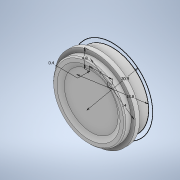
# Autodesk Inventor part: fingerprint sensor
Saved by Autodesk Inventor 2022 (Build 260153000, 153)
## iProperties
Created: 2022-06-08
Part Number: fingerprint sensor
Material: Generic
Document SubType Name: Modeling
Designer: alecw
Density: 1 g/cm^3
Appearance: Default
Author: alecw
Autodesk Inventor part; units mm, degrees
ref_plane "YZ Plane" through (0, 0, 0) normal (1, 0, 0) x (0, 1, 0)
ref_plane "XZ Plane" through (0, 0, 0) normal (0, 1, 0) x (-1, 0, 0)
ref_plane "XY Plane" through (0, 0, 0) normal (0, 0, 1) x (1, 0, 0)
sketch "Sketch1" plane through (0, 0, 0) normal (0, 0, 1) x (1, 0, 0)
  circle A0 centre (0, 0) radius 9.4
  circle A1 centre (0, 0) radius 10.45
  circle A2 centre (0, 0) radius 7
  line L0 (0, 0) -> (0, 1)
  line L1 (0, 1) -> (-5.6, 1)
  line L2 (-6, 1.4) -> (-6, 5.4)
  line L3 (-5.6, 5.8) -> (0, 5.8)
  arc A3 (-6, 1.4) -> (-5.6, 1) centre (-5.6, 1.4) ccw
  arc A4 (-5.6, 5.8) -> (-6, 5.4) centre (-5.6, 5.4) ccw
  line L4 (0, 1) -> (5.6, 1)
  line L5 (6, 1.4) -> (6, 5.4)
  line L6 (5.6, 5.8) -> (0, 5.8)
  arc A5 (5.6, 1) -> (6, 1.4) centre (5.6, 1.4) ccw
  arc A6 (6, 5.4) -> (5.6, 5.8) centre (5.6, 5.4) ccw
  point P0 (-6, 1)
  point P1 (-6, 5.8)
  dimension "d0" = 18.8
  dimension "d1" = 20.9
  dimension "d8" = 14
  dimension "d18" = 1
  dimension "d19" = 6
  dimension "d20" = 4.8
  dimension "d21" = 0.4
  constraints: 14 end point, 8 point on circle, 7 centre point, 6 symmetric about line, 4 point on line, 4 tangent, 3 coincident, 2 perpendicular, 2 vertical, 1 equal radius, 2 other
  measures "d0" diameter of A0
  measures "d1" diameter of A1
  measures "d8" diameter of A2
  measures "d18" distance of L0.start L0.end
  measures "d19" distance of L0.end point (-6, 1)
  measures "d20" distance of point (-6, 1) point (-6, 5.8)
  measures "d21" radius of A3
extrude "Extrusion1" add sketch "Sketch1" along normal blind 3.3 contours A0 | A2 L2 A3 L1 L4 A5 L5 | L5 A5 L4 L1 A3 L2 A2 L3 L6 | A2 L6 A6 L5 | L2 A4 L3 A2 | L6 L3 A2
extrude "Extrusion2" add sketch "Sketch1" along normal blind 1.2 from surface at 3.3 contours A0 | A1 | A2 L2 A3 L1 L4 A5 L5 | L5 A5 L4 L1 A3 L2 A2 L3 L6 | A2 L6 A6 L5 | L2 A4 L3 A2 | L6 L3 A2
extrude "Extrusion3" add sketch "Sketch1" along normal blind 1.7 from surface at 4.5 contours A0 | A2 L2 A3 L1 L4 A5 L5 | L5 A5 L4 L1 A3 L2 A2 L3 L6 | A2 L6 A6 L5 | L2 A4 L3 A2 | L6 L3 A2
extrude "Extrusion4" cut sketch "Sketch1" against normal blind 0.7 from surface at 6.2 contours A2 L2 A3 L1 L4 A5 L5 | L5 A5 L4 L1 A3 L2 A2 L3 L6 | L6 L3 A2
chamfer "Chamfer1" distance 0.7 angle 60 1 edges at (-7, 0, 6.2) measured on face at (-7, 0, 5.7)
chamfer "Chamfer2" distance 0.3 angle 45 1 edges at (-9.4, 0, 6.2)
body "Solid1"
